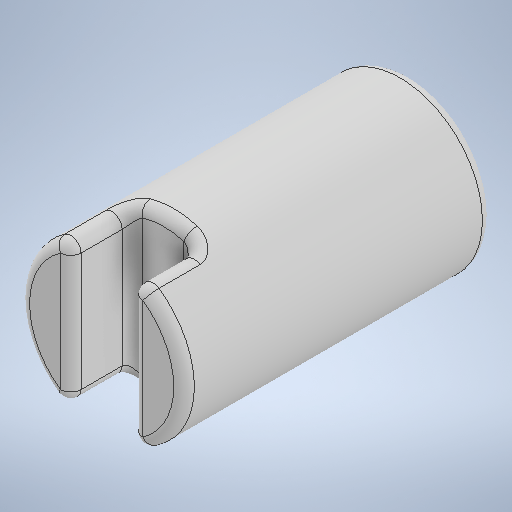
# Autodesk Inventor part: Locating Pin
Saved by Autodesk Inventor 2025.2 (Build 292293000, 293)
## iProperties
Created: 2025-02-07
Part Number: Locating Pin
Material: Generic
Document SubType Name: Modeling
Designer: eason
Density: 1 g/cm^3
Appearance: Default
Author: eason
Autodesk Inventor part; units mm, degrees
ref_plane "YZ Plane" through (0, 0, 0) normal (1, 0, 0) x (0, 1, 0)
ref_plane "XZ Plane" through (0, 0, 0) normal (0, 1, 0) x (-1, 0, 0)
ref_plane "XY Plane" through (0, 0, 0) normal (0, 0, 1) x (1, 0, 0)
sketch "Sketch1" plane through (0, 0, 0) normal (0, 0, 1) x (1, 0, 0)
  circle A0 centre (0, 0) radius 4
  dimension "d0" = 8
  constraints: 1 centre point, 1 coincident
  measures "d0" diameter of A0
extrude "Extrusion1" add sketch "Sketch1" along normal blind 15
sketch "Sketch2" plane through (0, 0, 15) normal (0, 0, 1) x (1, 0, 0)
  circle A0 centre (0, 0) radius 4 projected
  line L0 (0, -5.6) -> (0, 5.6) projected
  line L1 (1.5, -3.7081) -> (1.5, 3.7081)
  line L2 (-1.5, -3.7081) -> (-1.5, 3.7081)
  circle A1 centre (0, 0) radius 4 projected
  dimension "d5" = 3
  dimension "d6" = 1.5
  constraints: 4 end point, 4 point on circle, 2 parallel
  measures "d5" distance between parallel lines of L2 L1
  measures "d6" distance between parallel lines of L1 L0
extrude "Extrusion2" cut sketch "Sketch2" against normal blind 3 contours L1 A0 L0 | L0 A0 L2
fillet "Fillet1" radius 0.5 14 edges at (-1.5, 0, 15) (1.5, 0, 15) (-1.5, 0, 12) (1.5, 0, 12) (3.3166, -2.2361, 15) (3.3166, 2.2361, 15) (-4, 0, 15) (-1.5, -3.7081, 13.5) (-1.5, 3.7081, 13.5) (1.5, -3.7081, 13.5) (1.5, 3.7081, 13.5) (0, -4, 12) (0, 4, 12) (-4, 0, 0)
body "Solid1"
